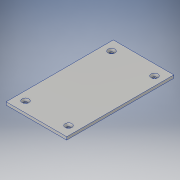
# Autodesk Inventor part: Piston Feed surface
Saved by Autodesk Inventor 2018.1 (Build 221171000, 171)
## iProperties
Created: 2013-10-18
Part Number: Piston Feed surface
Material: Aluminum 6061
Document SubType Name: Modeling
Designer: Gabriel Smolnycki
Mass: 135.122 g
Surface Area: 271.865 cm^2
Volume: 50.0452 cm^3
Density: 2.7 g/cm^3
Appearance: Aluminum - Flat
Author: Gabriel Smolnycki
Sending System: SolidWorks 2017
Last Author: Gabriel Smolnycki
Last Saved: 2017-09-14
Autodesk Inventor part; units mm, degrees
ref_plane "XZ Plane" through (0, 0, 0) normal (0, 1, 0) x (-1, 0, 0)
ref_plane "XY Plane" through (0, 0, 0) normal (0, 0, 1) x (1, 0, 0)
ref_plane "Work Plane1" through (-42.25, 0, 0) normal (1, 0, 0) x (0, 1, 0)
sketch "Sketch1" plane through (-42.25, 0, 0) normal (1, 0, 0) x (0, 1, 0)
  line L0 (0.064, -74.75) -> (0.064, 74.75)
  line L1 (-4, 74.75) -> (0.064, 74.75)
  line L2 (-4, -74.75) -> (0.064, -74.75)
  line L3 (-4, -74.75) -> (-4, 74.75)
  dimension "d31" = 4.064
  dimension "d32" = 149.5
  constraints: 8 end point, 2 horizontal, 2 vertical
  measures "d31" distance between parallel lines of L3 L0
  measures "d32" distance of L0.start L0.end
extrude "Extrusion2" add sketch "Sketch1" along normal blind 84.5
sketch "Sketch2" plane through (0, 0.064, 0) normal (0, 1, 0) x (-1, 0, 0)
  point P0 (-30, -60)
hole "Hole8" at (30, 0.064, -60) direction (0, -1, 0) diameter 4.5 depth 4.064 countersink diameter 9.4 countersink angle 90
sketch "Sketch3" plane through (0, 0.064, 0) normal (0, 1, 0) x (-1, 0, 0)
  point P0 (30, 60)
hole "Hole7" at (-30, 0.064, 60) direction (0, -1, 0) diameter 4.5 depth 4.064 countersink diameter 9.4 countersink angle 90
sketch "Sketch4" plane through (0, 0.064, 0) normal (0, 1, 0) x (-1, 0, 0)
  point P0 (-30, 60)
hole "Hole6" at (30, 0.064, 60) direction (0, -1, 0) diameter 4.5 depth 4.064 countersink diameter 9.4 countersink angle 90
sketch "Sketch5" plane through (0, 0.064, 0) normal (0, 1, 0) x (-1, 0, 0)
  point P0 (30, -60)
hole "Hole5" at (-30, 0.064, -60) direction (0, -1, 0) diameter 4.5 depth 4.064 countersink diameter 9.4 countersink angle 90
body "Solid3"
